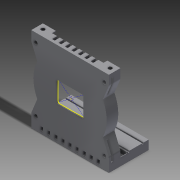
# Autodesk Inventor part: Nikon Base 02
Saved by Autodesk Inventor 2013 (Build 170138000, 138)
## iProperties
Created: 2014-04-13
Part Number: Nikon Base 02
Material: Generic
Document SubType Name: Modeling
Designer: spichelh
Density: 1 g/cm^3
Author: spichelh
Autodesk Inventor part; units mm, degrees
ref_plane "YZ Plane" through (0, 0, 0) normal (1, 0, 0) x (0, 1, 0)
ref_plane "XZ Plane" through (0, 0, 0) normal (0, 1, 0) x (-1, 0, 0)
ref_plane "XY Plane" through (0, 0, 0) normal (0, 0, 1) x (1, 0, 0)
sketch "Sketch1" plane through (0, 0, 0) normal (0, 0, 1) x (1, 0, 0)
  line L0 (0, -8.8929) -> (0, 44.5272) construction
  circle A0 centre (26.67, 24.765) radius 3.5 construction
  circle A1 centre (26.67, 24.765) radius 1.4
  line L1 (-0.1076, 0) -> (-29.2451, 0) construction
  line L2 (-21.59, -19.685) -> (-21.59, -28.575) construction
  circle A2 centre (-26.67, 24.765) radius 3.5 construction
  circle A3 centre (-26.67, 24.765) radius 1.4
  circle A4 centre (-26.67, -24.765) radius 1.4
  circle A5 centre (-26.67, -24.765) radius 3.5 construction
  circle A6 centre (26.67, -24.765) radius 1.4
  circle A7 centre (26.67, -24.765) radius 3.5 construction
  line L3 (-26.67, 24.765) -> (26.67, -24.765) construction
  line L4 (26.67, 24.765) -> (-26.67, -24.765) construction
  line L5 (-21.59, 19.685) -> (-21.59, 28.575) construction
  line L6 (21.59, -19.685) -> (21.59, -28.575) construction
  line L7 (21.59, 19.685) -> (21.59, 28.575) construction
  line L8 (-21.67, 30.575) -> (21.67, 30.575) construction
  line L9 (21.67, 30.575) -> (21.67, -25.765) construction
  line L10 (21.67, -25.765) -> (-21.67, -25.765) construction
  line L11 (-21.67, -25.765) -> (-21.67, 30.575) construction
  line L12 (-50.8, 28.575) -> (50.8, 28.575) construction
  line L13 (50.8, 28.575) -> (50.8, -28.575) construction
  line L14 (50.8, -28.575) -> (-50.8, -28.575) construction
  line L15 (-50.8, -28.575) -> (-50.8, 28.575) construction
  line L16 (-50.8, 28.575) -> (50.8, -28.575) construction
  line L17 (50.8, 28.575) -> (-50.8, -28.575) construction
  line L18 (-30.17, -29.575) -> (-30.17, -24.765)
  line L19 (30.17, -29.575) -> (30.17, -24.765)
  line L20 (-30.17, -29.575) -> (30.17, -29.575)
  line L21 (22.37, -28.575) -> (-22.37, -28.575)
  arc A8 (-29.9124, -23.447) -> (-30.17, -24.765) centre (-26.67, -24.765) ccw
  arc A9 (30.17, -24.765) -> (29.9124, -23.447) centre (26.67, -24.765) ccw
  circle A10 centre (26.67, 24.765) radius 1.4
  line L22 (30.17, 24.765) -> (30.17, 31.575)
  line L23 (-30.17, 31.575) -> (30.17, 31.575)
  line L24 (-30.17, 24.765) -> (-30.17, 31.575)
  line L25 (-22.37, 29.575) -> (22.37, 29.575)
  arc A11 (-30.17, 24.765) -> (-29.9124, 23.447) centre (-26.67, 24.765) ccw
  arc A12 (29.9124, 23.447) -> (30.17, 24.765) centre (26.67, 24.765) ccw
  circle A13 centre (0, 0) radius 28.5 construction
  line L26 (29.9124, -23.447) -> (25.5304, -12.6669)
  line L27 (29.9124, 23.447) -> (25.5304, 12.6669)
  arc A14 (25.5304, -12.6669) -> (25.5304, 12.6669) centre (0, 0) ccw
  line L28 (29.9124, 23.447) -> (26.67, 24.765) construction
  line L29 (-29.9124, -23.447) -> (-25.5304, -12.6669)
  line L30 (-29.9124, 23.447) -> (-25.5304, 12.6669)
  arc A15 (-25.5304, 12.6669) -> (-25.5304, -12.6669) centre (0, 0) ccw
  line L31 (22.37, 29.575) -> (22.37, -28.575)
  line L32 (-22.37, -28.575) -> (-22.37, 29.575)
  point P0 (0, 0)
  point P1 (0, 0)
  point P2 (0, 0)
  point P3 (24.8655, -21.7661)
  point P4 (0.1677, 29.575)
  point P5 (-23.17, 24.765)
  point P6 (-23.17, -24.765)
  point P7 (23.17, -24.765)
  point P8 (23.17, 24.765)
  point P9 (0, 0)
  point P10 (0, 0)
  point P11 (0, 0)
  dimension "d315" = 7
  dimension "d320" = 2.8
  dimension "d327" = 85
  dimension "d328" = 8.89
  dimension "d332" = 53.34
  dimension "d333" = 49.53
  dimension "d334" = 2.8
  dimension "d335" = 7
  dimension "d337" = 5.08
  dimension "d339" = 5
  dimension "d340" = 5
  dimension "d341" = 1
  dimension "d342" = 101.6
  dimension "d343" = 57.15
  dimension "d344" = 2
  dimension "d363" = 7
  dimension "d364" = 2.8
  dimension "d366" = 1
  dimension "d367" = 2
  dimension "d368" = 1
  dimension "d377" = 3.5
  dimension "d378" = 6.81
  dimension "d403" = 57
  dimension "d417" = 155
  dimension "d418" = 155
  dimension "d422" = 0.7
  dimension "d423" = 0.7
  constraints: 70 end point, 24 point on circle, 16 centre point, 15 symmetric about line, 7 coincident, 7 midpoint, 7 perpendicular, 6 parallel, 5 concentric, 5 tangent, 4 point on line, 3 horizontal, 2 horizontal alignment, 1 vertical alignment, 5 other
  measures "d315" diameter of A0
  measures "d320" diameter of A1
  measures "d328" distance of L2.start L2.end
  measures "d332" distance of A0.centre A2.centre
  measures "d333" distance of point (-26.67, -24.765) A2.centre
  measures "d334" diameter of A4
  measures "d335" diameter of A5
  measures "d337" distance from line of A4.centre L2
  measures "d339" distance from line of A0.centre L9
  measures "d340" distance from line of A2.centre L11
  measures "d341" distance from line of L10 A6.centre
  measures "d342" distance of L13.end L14.end
  measures "d343" distance of L12.end L13.end
  measures "d344" distance between parallel lines of L12 L8
  measures "d363" diameter of A2
  measures "d364" diameter of A3
  measures "d366" distance between parallel lines of L12 L25
  measures "d367" distance between parallel lines of L23 L25
  measures "d368" distance between parallel lines of L21 L20
  measures "d377" radius of A12
  measures "d378" distance of L22.start L22.end
  measures "d403" diameter of A13
  measures "d417" angle of L26 L3
  measures "d418" angle of L4 L27
  measures "d422" distance between parallel lines of L9 L31
  measures "d423" distance between parallel lines of L11 L32
extrude "Extrusion1" add sketch "Sketch1" along normal blind 9
sketch "Sketch14" plane through (0, 0, 9) normal (0, 0, 1) x (1, 0, 0)
  line L0 (50.88, 56.34) -> (5, 56.34) construction
  line L1 (-22.86, -0.81) -> (78.74, -0.81) construction
  line L2 (-22.86, 56.34) -> (-22.86, -0.81) construction
  line L3 (78.74, -0.81) -> (78.74, 56.34) construction
  circle A0 centre (26.67, 24.765) radius 1.4 projected
  arc A1 (-29.9124, -23.447) -> (-30.17, -24.765) centre (-26.67, -24.765) ccw projected
  line L4 (-30.17, -29.575) -> (30.17, -29.575) projected
  arc A2 (30.17, -24.765) -> (29.9124, -23.447) centre (26.67, -24.765) ccw projected
  line L5 (-27.94, 24.765) -> (26.67, -24.765) construction
  line L6 (-26.67, -24.765) -> (26.67, 24.765) construction
  circle A3 centre (0, 0) radius 23
  line L7 (27.3548, 30.2966) -> (-26.2048, 30.2966)
  line L8 (-26.67, -29.1989) -> (25.27, -29.1989)
  line L9 (30.17, 31.575) -> (-30.17, 31.575) projected
  line L10 (-26.2048, 30.2966) -> (-25.2211, 26.462)
  line L11 (-25.2211, 26.462) -> (-25.2211, 23)
  line L12 (-25.2211, 23) -> (-25.2211, 18.3922)
  line L13 (-25.2211, 18.3922) -> (-25.0819, 16.5883)
  line L14 (-25.1417, -26.7599) -> (-26.67, -29.1989)
  line L15 (25.27, -29.1989) -> (25.1417, -24.765)
  line L16 (25.1417, -24.765) -> (25.1912, -21.1)
  line L17 (25.1912, -21.1) -> (25.27, -15.2651)
  line L18 (25.27, -15.2651) -> (24.6585, -7.3445)
  line L19 (24.6585, -7.3445) -> (24.4818, 2.6027)
  line L20 (24.4818, 2.6027) -> (25.1533, 16.767)
  line L21 (25.1533, 16.767) -> (25.4405, 22.8257)
  line L22 (25.4405, 22.8257) -> (25.0053, 24.5219)
  line L23 (25.0053, 24.5219) -> (25.27, 26.707)
  line L24 (25.27, 26.707) -> (27.3548, 30.2966)
  line L25 (-30.17, 31.575) -> (-30.17, 24.765) projected
  line L26 (-25.1417, -26.7599) -> (-25.1417, -18.1825)
  line L27 (-25.1417, -18.1825) -> (-24.2585, 0.4493)
  line L28 (-24.2585, 0.4493) -> (-25.0819, 16.5883)
  dimension "d359" = 46
  constraints: 44 end point, 5 parallel, 3 collinear, 1 centre point, 1 midpoint, 1 perpendicular
  measures "d359" diameter of A3
extrude "Extrusion14" add sketch "Sketch14" against normal blind 2 contours L24 L23 L22 L21 L20 L19 L18 L17 L16 L15 L8 L14 L26 L27 L28 L13 L12 L11 L10 L7
sketch "Sketch17" plane through (0, 0, 7) normal (0, 0, -1) x (-1, 0, 0)
  line L0 (-9.4, 8.05) -> (9.4, 8.05)
  line L1 (10.4, 7.05) -> (10.4, -7.05)
  line L2 (9.4, -8.05) -> (-9.4, -8.05)
  line L3 (-10.4, -7.05) -> (-10.4, 7.05)
  line L4 (10.4, 8.05) -> (-10.4, -8.05) construction
  line L5 (10.4, -8.05) -> (-10.4, 8.05) construction
  circle A0 centre (0, 0) radius 23
  arc A1 (-9.4, 8.05) -> (-10.4, 7.05) centre (-9.4, 7.05) ccw
  arc A2 (-10.4, -7.05) -> (-9.4, -8.05) centre (-9.4, -7.05) ccw
  arc A3 (9.4, -8.05) -> (10.4, -7.05) centre (9.4, -7.05) ccw
  arc A4 (10.4, 7.05) -> (9.4, 8.05) centre (9.4, 7.05) ccw
  dimension "d111" = 20.8
  dimension "d112" = 16.1
  dimension "d115" = 1
  constraints: 12 end point, 8 point on circle, 8 point on line, 8 tangent, 5 centre point, 3 equal radius, 2 coincident, 2 parallel, 1 horizontal, 1 midpoint, 1 perpendicular
  measures "d111" distance of L5.start L4.end
  measures "d112" distance of L4.start L5.start
  measures "d115" radius of A1
extrude "Extrusion17" add sketch "Sketch17" against normal blind 2
sketch "Sketch26" plane through (0, 6, 0) normal (-1, 0, 0) x (0, 0, 1)
  line L0 (0, 43.53) -> (0, 0) projected
  line L1 (-1, 50.34) -> (0, 50.34) construction
  line L2 (-1, -6.81) -> (0, -6.81) construction
  line L3 (4, -6.81) -> (6, -6.81)
  line L4 (6, -6.81) -> (6, 50.34)
  line L5 (6, 50.34) -> (4, 50.34)
  line L6 (4, 50.34) -> (4, -6.81)
  point P0 (0, -6)
  dimension "d140" = 2
  dimension "d141" = 4
  constraints: 8 end point, 2 collinear, 2 parallel, 1 horizontal, 1 perpendicular
  measures "d140" distance of L5.end L4.end
  measures "d141" distance between parallel lines of L0 L6
extrude "Extrusion26" [suppressed]
sketch "Sketch27" plane through (55.88, 6, 0) normal (1, 0, 0) x (0, 0, -1)
  line L0 (1, -6.81) -> (0, -6.81) construction
  line L1 (1, 50.34) -> (0, 50.34) construction
  line L2 (-4, 50.34) -> (-6, 50.34)
  line L3 (-6, 50.34) -> (-6, -6.81)
  line L4 (-6, -6.81) -> (-4, -6.81)
  line L5 (-4, -6.81) -> (-4, 50.34)
  line L6 (0, -13) -> (0, -6) construction
  dimension "d146" = 2
  dimension "d147" = 4
  constraints: 8 end point, 2 collinear, 2 parallel, 1 horizontal, 1 perpendicular
  measures "d146" distance of L4.end L3.end
  measures "d147" distance between parallel lines of L6 L5
extrude "Extrusion27" [suppressed]
sketch "Sketch32" plane through (0, 0, 0) normal (0, 0, -1) x (-1, 0, 0)
  line L0 (-30.17, -34.575) -> (30.17, -34.575)
  line L1 (30.17, -34.575) -> (30.17, -28.575)
  line L2 (30.17, -28.575) -> (-30.17, -28.575)
  line L3 (-30.17, -28.575) -> (-30.17, -34.575)
  line L4 (30.17, -29.575) -> (-30.17, -29.575)
  circle A0 centre (-26.67, -24.765) radius 1.4 projected
  circle A1 centre (26.67, -24.765) radius 1.4 projected
  circle A2 centre (26.67, 24.765) radius 1.4 projected
  circle A3 centre (-26.67, 24.765) radius 1.4 projected
  line L5 (-30.17, 31.575) -> (30.17, 31.575) projected
  line L6 (-30.17, 24.765) -> (-30.17, 31.575) projected
  arc A4 (-29.9124, -23.447) -> (-30.17, -24.765) centre (-26.67, -24.765) ccw projected
  line L7 (-30.17, -29.575) -> (-30.17, -24.765) projected
  line L8 (30.17, -29.575) -> (-30.17, -29.575) projected
  line L9 (30.17, -24.765) -> (30.17, -29.575) projected
  arc A5 (30.17, -24.765) -> (29.9124, -23.447) centre (26.67, -24.765) ccw projected
  line L10 (0, -34.575) -> (0, -36.1591) construction
  line L11 (0, -31.3897) -> (0, -27.0731) construction
  line L12 (-30.17, -29.575) -> (-30.17, -24.765) projected
  arc A6 (29.9124, 23.447) -> (30.17, 24.765) centre (26.67, 24.765) ccw projected
  line L13 (30.17, 31.575) -> (30.17, 24.765) projected
  arc A7 (-30.17, 24.765) -> (-29.9124, 23.447) centre (-26.67, 24.765) ccw projected
  line L14 (25.5304, -12.6669) -> (29.9124, -23.447) projected
  arc A8 (25.5304, -12.6669) -> (25.5304, 12.6669) centre (0, 0) ccw projected
  line L15 (29.9124, 23.447) -> (25.5304, 12.6669) projected
  line L16 (-25.5304, 12.6669) -> (-29.9124, 23.447) projected
  arc A9 (-25.5304, 12.6669) -> (-25.5304, -12.6669) centre (0, 0) ccw projected
  line L17 (-29.9124, -23.447) -> (-25.5304, -12.6669) projected
  dimension "d180" = 6
  dimension "d432" = 1
  constraints: 14 end point, 3 collinear, 3 parallel, 1 horizontal, 1 midpoint, 1 perpendicular
  measures "d180" distance between parallel lines of L0 L2
  measures "d432" distance between parallel lines of L4 L2
extrude "Extrusion32" add sketch "Sketch32" along normal blind 22 and the other way blind 1.5 contours L3 L4 L1 L0 | L3 L2 L1 L4
sketch "Sketch35" plane through (-30.17, -34.575, -22) normal (0, -1, 0) x (1, 0, 0)
  line L0 (60.34, 33) -> (0, 33)
  line L1 (0, 33) -> (60.34, 0) construction
  line L2 (60.34, 33) -> (0, 0) construction
  line L3 (30.17, 16.5) -> (30.17, -14.8721) construction
  circle A0 centre (30.17, 6.5) radius 3.175
  circle A1 centre (30.17, 18.5) radius 3.175
  line L4 (0, 23.5) -> (60.34, 23.5) projected
  dimension "d194" = 6.35
  dimension "d195" = 10
  dimension "d196" = 6.35
  dimension "d197" = 2
  dimension "d369" = 5
  constraints: 8 end point, 2 centre point, 2 point on line, 2 vertical alignment, 1 horizontal, 1 midpoint, 1 perpendicular
  measures "d194" diameter of A0
  measures "d195" distance of L3.start A0.centre
  measures "d196" diameter of A1
  measures "d197" distance of L3.start A1.centre
  measures "d369" distance from line of A1.centre L4
extrude "Extrusion34" cut sketch "Sketch35" against normal blind 10
sketch "Sketch37" plane through (52.88, -28.575, 0) normal (0, 1, 0) x (1, 0, 0)
  line L0 (-49.88, -1.5) -> (-49.88, 0) projected
  line L1 (3, -1.5) -> (-52.88, -1.5) projected
  line L2 (0, -1.5) -> (-49.88, -1.5)
  line L3 (-49.88, -1.5) -> (-49.88, 0)
  line L4 (-49.88, 0) -> (0, 0)
  line L5 (0, 0) -> (0, -1.5)
  constraints: 8 end point, 2 parallel, 1 horizontal, 1 perpendicular
extrude "Extrusion36" [suppressed]
sketch "Sketch38" plane through (0, 0, 7) normal (0, 0, -1) x (-1, 0, 0)
  arc A0 (-10.4, -7.05) -> (-9.4, -8.05) centre (-9.4, -7.05) ccw projected
  line L0 (-10.4, -7.05) -> (-10.4, 7.05) projected
  arc A1 (-9.4, 8.05) -> (-10.4, 7.05) centre (-9.4, 7.05) ccw projected
  line L1 (-9.4, 8.05) -> (9.4, 8.05) projected
  arc A2 (10.4, 7.05) -> (9.4, 8.05) centre (9.4, 7.05) ccw projected
  line L2 (10.4, 7.05) -> (10.4, -7.05) projected
  arc A3 (9.4, -8.05) -> (10.4, -7.05) centre (9.4, -7.05) ccw projected
  line L3 (9.4, -8.05) -> (-9.4, -8.05) projected
  line L4 (9.4, 7.05) -> (-9.4, -7.05) construction
  line L5 (9.4, -7.05) -> (-9.4, 7.05) construction
  line L6 (-21.665, 19.44) -> (21.665, 19.44)
  line L7 (21.665, 19.44) -> (21.665, -19.44)
  line L8 (21.665, -19.44) -> (-21.665, -19.44)
  line L9 (-21.665, -19.44) -> (-21.665, 19.44)
  line L10 (21.665, -19.44) -> (-21.665, 19.44) construction
  line L11 (-21.665, -19.44) -> (21.665, 19.44) construction
  point P0 (0, 0)
  point P1 (0, 0)
  dimension "d209" = 38.88
  dimension "d211" = 43.33
  constraints: 16 end point, 3 midpoint, 2 parallel, 1 horizontal, 1 perpendicular
  measures "d209" distance of L8.end L6.start
  measures "d211" distance of L6.start L6.end
extrude "Extrusion37" cut sketch "Sketch38" against normal blind 1
sketch "Sketch39" plane through (0, 0, 8) normal (0, 0, -1) x (-1, 0, 0)
  line L0 (-9.4, -8.05) -> (9.4, -8.05) projected
  arc A0 (-10.4, -7.05) -> (-9.4, -8.05) centre (-9.4, -7.05) ccw projected
  line L1 (-10.4, 7.05) -> (-10.4, -7.05) projected
  arc A1 (-9.4, 8.05) -> (-10.4, 7.05) centre (-9.4, 7.05) ccw projected
  line L2 (9.4, 8.05) -> (-9.4, 8.05) projected
  arc A2 (10.4, 7.05) -> (9.4, 8.05) centre (9.4, 7.05) ccw projected
  line L3 (10.4, -7.05) -> (10.4, 7.05) projected
  arc A3 (9.4, -8.05) -> (10.4, -7.05) centre (9.4, -7.05) ccw projected
  line L4 (-21.665, 19.44) -> (21.665, 19.44) projected
  line L5 (-21.665, -19.44) -> (-21.665, 19.44) projected
  line L6 (21.665, -19.44) -> (-21.665, -19.44) projected
  line L7 (21.665, 19.44) -> (21.665, -19.44) projected
  line L8 (9.4, 7.05) -> (-9.4, -7.05) construction
  line L9 (-9.4, 7.05) -> (9.4, -7.05) construction
  point P0 (0, 0)
  point P1 (0, 0)
  constraints: 4 end point, 1 midpoint
sketch "Sketch40" plane through (0, 0, 9) normal (0, 0, 1) x (1, 0, 0)
  line L0 (-20, 31.575) -> (20, 31.575)
  line L1 (20, 31.575) -> (20, 33.575)
  line L2 (20, 33.575) -> (-20, 33.575)
  line L3 (-20, 33.575) -> (-20, 31.575)
  line L4 (30.17, 31.575) -> (-30.17, 31.575) projected
  line L5 (0, 33.575) -> (0, 37.7765) construction
  line L6 (0, 31.575) -> (0, 28.075) construction
  dimension "d216" = 2
  dimension "d217" = 40
  constraints: 12 end point, 3 collinear, 2 midpoint, 2 parallel, 1 horizontal, 1 perpendicular, 1 vertical
  measures "d216" distance of L2.end L0.start
  measures "d217" distance between parallel lines of L3 L1
extrude "Extrusion38" [suppressed]
sketch "Sketch43" plane through (-30.17, 31.575, 0) normal (0, 1, 0) x (1, 0, 0)
  line L0 (47.17, 21) -> (13.17, 21)
  line L1 (13.17, 26) -> (13.17, 21)
  line L2 (47.17, 26) -> (13.17, 26)
  line L3 (47.17, 26) -> (47.17, 21)
  line L4 (14.17, 27) -> (16.17, 27)
  line L5 (16.17, 27) -> (16.17, 22)
  line L6 (16.17, 22) -> (14.17, 22)
  line L7 (14.17, 22) -> (14.17, 27)
  line L8 (19.17, 27) -> (21.17, 27)
  line L9 (21.17, 27) -> (21.17, 22)
  line L10 (21.17, 22) -> (19.17, 22)
  line L11 (19.17, 22) -> (19.17, 27)
  line L12 (24.17, 27) -> (26.17, 27)
  line L13 (26.17, 27) -> (26.17, 22)
  line L14 (26.17, 22) -> (24.17, 22)
  line L15 (24.17, 22) -> (24.17, 27)
  line L16 (29.17, 27) -> (31.17, 27)
  line L17 (31.17, 27) -> (31.17, 22)
  line L18 (31.17, 22) -> (29.17, 22)
  line L19 (29.17, 22) -> (29.17, 27)
  line L20 (34.17, 27) -> (36.17, 27)
  line L21 (36.17, 27) -> (36.17, 22)
  line L22 (36.17, 22) -> (34.17, 22)
  line L23 (34.17, 22) -> (34.17, 27)
  line L24 (39.17, 27) -> (41.17, 27)
  line L25 (41.17, 27) -> (41.17, 22)
  line L26 (41.17, 22) -> (39.17, 22)
  line L27 (39.17, 22) -> (39.17, 27)
  line L28 (44.17, 27) -> (46.17, 27)
  line L29 (46.17, 27) -> (46.17, 22)
  line L30 (46.17, 22) -> (44.17, 22)
  line L31 (44.17, 22) -> (44.17, 27)
  line L32 (10.17, 39.892) -> (10.17, -9)
  line L33 (50.17, 39.3269) -> (50.17, -9)
  line L34 (10.17, 10) -> (50.17, 10) construction
  line L35 (14.17, -7) -> (16.17, -7)
  line L36 (16.17, -7) -> (16.17, -2)
  line L37 (16.17, -2) -> (14.17, -2)
  line L38 (14.17, -2) -> (14.17, -7)
  line L39 (21.17, -7) -> (21.17, -2)
  line L40 (19.17, -7) -> (21.17, -7)
  line L41 (21.17, -2) -> (19.17, -2)
  line L42 (26.17, -7) -> (26.17, -2)
  line L43 (24.17, -7) -> (26.17, -7)
  line L44 (24.17, -2) -> (24.17, -7)
  line L45 (26.17, -2) -> (24.17, -2)
  line L46 (31.17, -7) -> (31.17, -2)
  line L47 (29.17, -7) -> (31.17, -7)
  line L48 (29.17, -2) -> (29.17, -7)
  line L49 (31.17, -2) -> (29.17, -2)
  line L50 (36.17, -7) -> (36.17, -2)
  line L51 (34.17, -7) -> (36.17, -7)
  line L52 (34.17, -2) -> (34.17, -7)
  line L53 (36.17, -2) -> (34.17, -2)
  line L54 (41.17, -7) -> (41.17, -2)
  line L55 (39.17, -7) -> (41.17, -7)
  line L56 (39.17, -2) -> (39.17, -7)
  line L57 (41.17, -2) -> (39.17, -2)
  line L58 (46.17, -7) -> (46.17, -2)
  line L59 (44.17, -7) -> (46.17, -7)
  line L60 (44.17, -2) -> (44.17, -7)
  line L61 (46.17, -2) -> (44.17, -2)
  line L62 (19.17, -2) -> (19.17, -7)
  line L63 (50.17, -9) -> (10.17, -9)
  line L64 (50.17, -9) -> (40, -9)
  line L65 (60.34, -9) -> (0, -9) projected
  line L66 (60.34, 0) -> (60.34, -9) projected
  line L67 (30.17, -9) -> (30.17, -4.5) construction
  line L68 (30.17, -9) -> (30.17, 3.8143) construction
  point P0 (0, 27)
  point P1 (50.17, 39.3269)
  dimension "d233" = 1
  dimension "d234" = 1
  dimension "d235" = 2
  dimension "d236" = 1
  dimension "d239" = 5
  dimension "d295" = 3
  dimension "d296" = 3
  dimension "d297" = 1
  dimension "d298" = 5
  dimension "d299" = 19
  dimension "d370" = 2
  dimension "d371" = 4
  dimension "d372" = 4
  dimension "d447" = 40
  constraints: 132 end point, 28 symmetric about line, 4 collinear, 3 horizontal, 3 parallel, 2 midpoint, 1 perpendicular, 1 point on line, 52 other
  measures "d233" distance between parallel lines of L2 L4
  measures "d234" distance between parallel lines of L0 L6
  measures "d235" distance between parallel lines of L7 L5
  measures "d236" distance between parallel lines of L7 L1
  measures "d239" distance of L4.end L9.start
  measures "d295" distance between parallel lines of L32 L1
  measures "d297" distance between parallel lines of L3 L29
  measures "d298" distance between parallel lines of L8 L10
  measures "d299" distance between parallel lines of L63 L34
  measures "d370" distance between parallel lines of L64 L40
  measures "d372" distance between parallel lines of L32 L38
extrude "Extrusion41" cut sketch "Sketch43" against normal blind 5 contours L29 L30 L31 L2 | L2 L31 L28 L29 | L7 L4 L5 L2 | L2 L5 L6 L7 | L25 L26 L27 L2 | L2 L27 L24 L25 | L11 L8 L9 L2 | L2 L9 L10 L11 | L21 L22 L23 L2 | L2 L23 L20 L21 | L15 L12 L13 L2 | L2 L13 L14 L15 | L17 L18 L19 L2 | L2 L19 L16 L17 | L38 L37 L36 L35 | L40 L62 L41 L39 | L43 L44 L45 L42 | L47 L48 L49 L46 | L51 L52 L53 L50 | L55 L56 L57 L54 | L59 L60 L61 L58
sketch "Sketch44" plane through (-24.8655, -28.575, 0) normal (0, 1, 0) x (1, 0, 0)
  line L0 (49.88, -7.5) -> (0, -7.5)
  line L1 (0, -7.5) -> (0, 0)
  line L2 (0, 0) -> (49.88, 0)
  line L3 (49.88, -7.5) -> (49.88, 0)
  line L4 (2, -1) -> (4, -1)
  line L5 (4, -1) -> (4, -6.5)
  line L6 (4, -6.5) -> (2, -6.5)
  line L7 (2, -6.5) -> (2, -1)
  line L8 (7.5, -1) -> (9.5, -1)
  line L9 (9.5, -1) -> (9.5, -6.5)
  line L10 (9.5, -6.5) -> (7.5, -6.5)
  line L11 (7.5, -6.5) -> (7.5, -1)
  line L12 (13, -1) -> (15, -1)
  line L13 (15, -1) -> (15, -6.5)
  line L14 (15, -6.5) -> (13, -6.5)
  line L15 (13, -6.5) -> (13, -1)
  line L16 (18.5, -1) -> (20.5, -1)
  line L17 (20.5, -1) -> (20.5, -6.5)
  line L18 (20.5, -6.5) -> (18.5, -6.5)
  line L19 (18.5, -6.5) -> (18.5, -1)
  line L20 (24, -1) -> (26, -1)
  line L21 (26, -1) -> (26, -6.5)
  line L22 (26, -6.5) -> (24, -6.5)
  line L23 (24, -6.5) -> (24, -1)
  line L24 (29.5, -1) -> (31.5, -1)
  line L25 (31.5, -1) -> (31.5, -6.5)
  line L26 (31.5, -6.5) -> (29.5, -6.5)
  line L27 (29.5, -6.5) -> (29.5, -1)
  line L28 (35, -1) -> (37, -1)
  line L29 (37, -1) -> (37, -6.5)
  line L30 (37, -6.5) -> (35, -6.5)
  line L31 (35, -6.5) -> (35, -1)
  line L32 (40.5, -1) -> (42.5, -1)
  line L33 (42.5, -1) -> (42.5, -6.5)
  line L34 (42.5, -6.5) -> (40.5, -6.5)
  line L35 (40.5, -6.5) -> (40.5, -1)
  line L36 (46, -1) -> (48, -1)
  line L37 (48, -1) -> (48, -6.5)
  line L38 (48, -6.5) -> (46, -6.5)
  line L39 (46, -6.5) -> (46, -1)
  point P0 (0, -9)
  dimension "d247" = 1
  dimension "d248" = 1
  dimension "d249" = 2
  dimension "d250" = 2
  dimension "d253" = 5.5
  dimension "d260" = 1.88
  constraints: 80 end point, 2 horizontal, 2 parallel, 1 perpendicular, 64 other
  measures "d247" distance between parallel lines of L2 L4
  measures "d248" distance between parallel lines of L0 L6
  measures "d249" distance between parallel lines of L7 L5
  measures "d250" distance between parallel lines of L1 L7
  measures "d253" distance of L4.end L9.start
  measures "d260" distance between parallel lines of L37 L3
extrude "Extrusion42" cut sketch "Sketch44" against normal blind 5 contours L4 L5 L6 L7 | L8 L9 L10 L11 | L12 L13 L14 L15 | L16 L17 L18 L19 | L20 L21 L22 L23 | L24 L25 L26 L27 | L28 L29 L30 L31 | L32 L33 L34 L35 | L36 L37 L38 L39
sketch "Sketch46" plane through (-20, 33.575, 15) normal (0, 1, 0) x (1, 0, 0)
  circle A0 centre (4, 36) radius 1.7
  circle A1 centre (36, 36) radius 1.7
  line L0 (36, 36) -> (4, 36) construction
  circle A2 centre (36, 4) radius 1.7
  line L1 (0, 40) -> (0, 0) projected
  line L2 (40, 0) -> (0, 0) projected
  line L3 (40, 40) -> (40, 0) projected
  line L4 (0, 40) -> (40, 40) projected
  line L5 (40, 20) -> (0, 20) construction
  line L6 (20, 40) -> (20, 0) construction
  line L7 (36, 4) -> (36, 36) construction
  circle A3 centre (4, 4) radius 1.7
  point P0 (20, 36)
  point P1 (36, 20)
  dimension "d275" = 3.4
  dimension "d277" = 3.4
  dimension "d278" = 32
  dimension "d279" = 32
  dimension "d294" = 3.4
  constraints: 8 end point, 6 midpoint, 4 centre point, 2 point on line, 1 horizontal, 1 symmetric about line, 1 other
  measures "d275" diameter of A0
  measures "d277" diameter of A1
  measures "d278" distance of L0.start L0.end
  measures "d279" distance of L7.start L0.start
  measures "d294" diameter of A2
extrude "Extrusion44" [suppressed]
sketch "Sketch49" plane through (0, 0, 0) normal (0, 0, -1) x (-1, 0, 0)
  line L0 (0, 55.53) -> (0, 58.53) projected
  line L1 (-55.88, 58.53) -> (0, 58.53)
  line L2 (0, 58.53) -> (0, 56.53)
  line L3 (0, 56.53) -> (-55.88, 56.53)
  line L4 (-55.88, 56.53) -> (-55.88, 58.53)
  constraints: 8 end point, 2 parallel, 1 horizontal, 1 perpendicular, 1 point on line
extrude "Extrusion46" [suppressed]
sketch "Sketch51" plane through (0, 0, 7) normal (0, 0, -1) x (-1, 0, 0)
  line L0 (21.665, -19.44) -> (-21.665, -19.44) projected
  line L1 (-3, -2.5) -> (-52.88, -2.5) projected
  line L2 (-37.44, -2.5) -> (-35.44, -2.5)
  line L3 (-35.44, -2.5) -> (-35.44, 0.5)
  line L4 (-35.44, 0.5) -> (-37.44, 0.5)
  line L5 (-37.44, 0.5) -> (-37.44, -2.5)
  line L6 (-27.94, -2.5) -> (-27.94, -19.44) construction
  line L7 (-31.94, -2.5) -> (-29.94, -2.5)
  line L8 (-29.94, -2.5) -> (-29.94, 0.5)
  line L9 (-29.94, 0.5) -> (-31.94, 0.5)
  line L10 (-31.94, 0.5) -> (-31.94, -2.5)
  line L11 (-26.44, -2.5) -> (-24.44, -2.5)
  line L12 (-24.44, -2.5) -> (-24.44, 0.5)
  line L13 (-24.44, 0.5) -> (-26.44, 0.5)
  line L14 (-26.44, 0.5) -> (-26.44, -2.5)
  line L15 (-20.94, -2.5) -> (-18.94, -2.5)
  line L16 (-18.94, -2.5) -> (-18.94, 0.5)
  line L17 (-18.94, 0.5) -> (-20.94, 0.5)
  line L18 (-20.94, 0.5) -> (-20.94, -2.5)
  point P0 (0, 0)
  dimension "d300" = 0
  dimension "d301" = 2
  dimension "d302" = 3
  dimension "d303" = 15
  dimension "d308" = 5.5
  constraints: 34 end point, 2 horizontal, 2 parallel, 1 midpoint, 1 perpendicular, 1 point on line, 24 other
  measures "d300" distance between parallel lines of L2 L1
  measures "d301" distance of L2.start L2.end
  measures "d302" distance between parallel lines of L4 L2
  measures "d303" diameter of L3 L6
  measures "d308" distance of L3.end L9.start
extrude "Extrusion48" [suppressed]
sketch "Sketch52" plane through (0, 0, 1.5) normal (0, 0, 1) x (1, 0, 0)
  line L0 (-30.17, -34.575) -> (30.17, -34.575) projected
  line L1 (30.17, -34.575) -> (30.17, -29.575) projected
  line L2 (-30.17, -29.575) -> (30.17, -29.575) projected
  line L3 (-30.17, -29.575) -> (-30.17, -34.575) projected
  line L4 (-30.17, -34.575) -> (30.17, -34.575) projected
  line L5 (30.17, -34.575) -> (30.17, -29.575) projected
  line L6 (-30.17, -29.575) -> (-22.8655, -29.575) projected
  line L7 (-30.17, -29.575) -> (-30.17, -34.575) projected
  line L8 (15.6345, -33.575) -> (15.6345, -29.575) projected
  line L9 (12.1345, -29.575) -> (15.6345, -29.575) projected
  line L10 (12.1345, -29.575) -> (12.1345, -33.575) projected
  line L11 (12.1345, -33.575) -> (10.1345, -33.575) projected
  line L12 (10.1345, -33.575) -> (10.1345, -29.575) projected
  line L13 (6.6345, -29.575) -> (10.1345, -29.575) projected
  line L14 (6.6345, -29.575) -> (6.6345, -33.575) projected
  line L15 (6.6345, -33.575) -> (4.6345, -33.575) projected
  line L16 (4.6345, -33.575) -> (4.6345, -29.575) projected
  line L17 (1.1345, -29.575) -> (4.6345, -29.575) projected
  line L18 (1.1345, -29.575) -> (1.1345, -33.575) projected
  line L19 (1.1345, -33.575) -> (-0.8655, -33.575) projected
  line L20 (-0.8655, -33.575) -> (-0.8655, -29.575) projected
  line L21 (-4.3655, -29.575) -> (-0.8655, -29.575) projected
  line L22 (-4.3655, -29.575) -> (-4.3655, -33.575) projected
  line L23 (-4.3655, -33.575) -> (-6.3655, -33.575) projected
  line L24 (-6.3655, -33.575) -> (-6.3655, -29.575) projected
  line L25 (-9.8655, -29.575) -> (-9.8655, -33.575) projected
  line L26 (-9.8655, -33.575) -> (-11.8655, -33.575) projected
  line L27 (-11.8655, -33.575) -> (-11.8655, -29.575) projected
  line L28 (-15.3655, -29.575) -> (-11.8655, -29.575) projected
  line L29 (-15.3655, -29.575) -> (-15.3655, -33.575) projected
  line L30 (-15.3655, -33.575) -> (-17.3655, -33.575) projected
  line L31 (-17.3655, -33.575) -> (-17.3655, -29.575) projected
  line L32 (-20.8655, -29.575) -> (-17.3655, -29.575) projected
  line L33 (-20.8655, -29.575) -> (-20.8655, -33.575) projected
  line L34 (-20.8655, -33.575) -> (-22.8655, -33.575) projected
  line L35 (-22.8655, -33.575) -> (-22.8655, -29.575) projected
  line L36 (23.1345, -29.575) -> (30.17, -29.575) projected
  line L37 (23.1345, -29.575) -> (23.1345, -33.575) projected
  line L38 (23.1345, -33.575) -> (21.1345, -33.575) projected
  line L39 (21.1345, -33.575) -> (21.1345, -29.575) projected
  line L40 (17.6345, -29.575) -> (21.1345, -29.575) projected
  line L41 (17.6345, -29.575) -> (17.6345, -33.575) projected
  line L42 (17.6345, -33.575) -> (15.6345, -33.575) projected
  line L43 (-9.8655, -29.575) -> (-6.3655, -29.575) projected
  point P0 (0, 0)
extrude "Extrusion49" add sketch "Sketch52" along normal blind 7.5
sketch "Sketch54" plane through (0, 0, 9) normal (0, 0, 1) x (1, 0, 0)
  line L0 (-30.17, -24.765) -> (-30.17, -34.575) projected
  line L1 (-30.17, -34.575) -> (30.17, -34.575) projected
  line L2 (30.17, -34.575) -> (30.17, -24.765) projected
  line L3 (-23, -29.575) -> (-21, -29.575)
  line L4 (-21, -29.575) -> (-21, -32.575)
  line L5 (-21, -32.575) -> (-23, -32.575)
  line L6 (-23, -32.575) -> (-23, -29.575)
  line L7 (-17.5, -29.575) -> (-15.5, -29.575)
  line L8 (-15.5, -29.575) -> (-15.5, -32.575)
  line L9 (-15.5, -32.575) -> (-17.5, -32.575)
  line L10 (-17.5, -32.575) -> (-17.5, -29.575)
  line L11 (-12, -29.575) -> (-10, -29.575)
  line L12 (-10, -29.575) -> (-10, -32.575)
  line L13 (-10, -32.575) -> (-12, -32.575)
  line L14 (-12, -32.575) -> (-12, -29.575)
  line L15 (-6.5, -29.575) -> (-4.5, -29.575)
  line L16 (-4.5, -29.575) -> (-4.5, -32.575)
  line L17 (-4.5, -32.575) -> (-6.5, -32.575)
  line L18 (-6.5, -32.575) -> (-6.5, -29.575)
  line L19 (-1, -29.575) -> (1, -29.575)
  line L20 (1, -29.575) -> (1, -32.575)
  line L21 (1, -32.575) -> (-1, -32.575)
  line L22 (-1, -32.575) -> (-1, -29.575)
  line L23 (4.5, -29.575) -> (6.5, -29.575)
  line L24 (6.5, -29.575) -> (6.5, -32.575)
  line L25 (6.5, -32.575) -> (4.5, -32.575)
  line L26 (4.5, -32.575) -> (4.5, -29.575)
  line L27 (10, -29.575) -> (12, -29.575)
  line L28 (12, -29.575) -> (12, -32.575)
  line L29 (12, -32.575) -> (10, -32.575)
  line L30 (10, -32.575) -> (10, -29.575)
  line L31 (15.5, -29.575) -> (17.5, -29.575)
  line L32 (17.5, -29.575) -> (17.5, -32.575)
  line L33 (17.5, -32.575) -> (15.5, -32.575)
  line L34 (15.5, -32.575) -> (15.5, -29.575)
  line L35 (21, -29.575) -> (23, -29.575)
  line L36 (23, -29.575) -> (23, -32.575)
  line L37 (23, -32.575) -> (21, -32.575)
  line L38 (21, -32.575) -> (21, -29.575)
  point P0 (0, 0)
  point P1 (-30.17, -29.575)
  point P2 (30.17, -29.575)
  dimension "d379" = 2
  dimension "d380" = 3
  dimension "d383" = 5.5
  dimension "d388" = 2
  dimension "d389" = 7.17
  dimension "d390" = 7.17
  constraints: 72 end point, 2 horizontal, 2 parallel, 1 collinear, 1 perpendicular, 63 other
  measures "d379" distance of L4.end L5.end
  measures "d380" distance of L3.end L4.end
  measures "d383" distance of L3.start L7.start
  measures "d388" distance between parallel lines of L5 L1
  measures "d389" distance between parallel lines of L0 L6
  measures "d390" distance between parallel lines of L2 L36
extrude "Extrusion51" cut sketch "Sketch54" against normal blind 8
sketch "Sketch55" plane through (0, 0, 0) normal (0, 0, -1) x (-1, 0, 0)
  line L0 (-20, 31.575) -> (20, 31.575) projected
  line L1 (-20, 31.575) -> (20, 31.575)
  line L2 (20, 31.575) -> (20, 29.575)
  line L3 (20, 29.575) -> (-20, 29.575)
  line L4 (-20, 29.575) -> (-20, 31.575)
  line L5 (-20, 33.575) -> (-20, 31.575) projected
  line L6 (20, 31.575) -> (20, 33.575) projected
  point P0 (-16, 31.575)
  point P1 (0, 0)
  dimension "d395" = 2
  constraints: 8 end point, 2 collinear, 2 parallel, 1 horizontal, 1 perpendicular, 1 point on line
  measures "d395" distance of L3.end L1.start
extrude "Extrusion52" cut sketch "Sketch55" against normal blind 3
sketch "Sketch56" plane through (0, 0, 0) normal (0, 0, -1) x (-1, 0, 0)
  line L0 (-20, 29.575) -> (-20, 31.575) projected
  line L1 (-30.17, 31.575) -> (-20, 31.575) projected
  line L2 (20, 29.575) -> (22.37, 29.575) projected
  line L3 (-22, 30.575) -> (21.185, 30.575)
  line L4 (21.185, 30.575) -> (21.185, 29.575)
  line L5 (21.185, 29.575) -> (-22, 29.575)
  line L6 (-22, 29.575) -> (-22, 30.575)
  point P0 (23.17, 29.575)
  point P1 (0, 0)
  dimension "d397" = 2
  dimension "d398" = 1
  constraints: 8 end point, 2 parallel, 1 horizontal, 1 midpoint, 1 perpendicular
  measures "d397" distance between parallel lines of L6 L0
  measures "d398" distance between parallel lines of L1 L3
extrude "Extrusion53" cut sketch "Sketch56" against normal blind 3
sketch "Sketch57" plane through (0, 0, 0) normal (0, 0, -1) x (-1, 0, 0)
  line L0 (-23.4203, 26.5752) -> (-29.9199, 26.5748) construction
  line L1 (-29.9199, 26.5748) -> (-30.1702, 28.5748) construction
  line L2 (-30.1702, 28.5748) -> (-30.1703, 29.9748) construction
  arc A0 (-29.5703, 30.5748) -> (-30.1703, 29.9748) centre (-29.5703, 29.9748) ccw construction
  line L3 (-29.5703, 30.5748) -> (-23.7703, 30.5752) construction
  arc A1 (-23.1703, 29.9752) -> (-23.7703, 30.5752) centre (-23.7703, 29.9752) ccw construction
  line L4 (-23.1703, 29.9752) -> (-23.1702, 28.5752) construction
  line L5 (-23.1702, 28.5752) -> (-23.4203, 26.5752) construction
  line L6 (20, 31.575) -> (20, 30.575) projected
  line L7 (0, 19.4123) -> (0, 6.0259) construction
  line L8 (30.17, 31.575) -> (-20, 31.575) projected
  line L9 (-29.0703, 30.6752) -> (-24.2699, 30.6752)
  line L10 (-29.5075, 26.4752) -> (-23.8327, 26.4752)
  line L11 (-29.5075, 26.4752) -> (-29.7703, 28.5748)
  line L12 (-29.7703, 29.9752) -> (-29.7703, 28.5748)
  arc A2 (-29.0703, 30.6752) -> (-29.7703, 29.9752) centre (-29.0703, 29.9752) ccw
  line L13 (-30.1702, 28.5748) -> (-29.2504, 28.5748) construction
  line L14 (-26.6701, 26.575) -> (-26.6701, 28.0459) construction
  line L15 (-23.8327, 26.4752) -> (-23.5699, 28.5748)
  line L16 (-23.5699, 29.9752) -> (-23.5699, 28.5748)
  arc A3 (-23.5699, 29.9752) -> (-24.2699, 30.6752) centre (-24.2699, 29.9752) ccw
  line L17 (29.0703, 30.6752) -> (24.2699, 30.6752)
  line L18 (29.5075, 26.4752) -> (23.8327, 26.4752)
  line L19 (29.5075, 26.4752) -> (29.7703, 28.5748)
  line L20 (29.7703, 29.9752) -> (29.7703, 28.5748)
  arc A4 (29.7703, 29.9752) -> (29.0703, 30.6752) centre (29.0703, 29.9752) ccw
  arc A5 (24.2699, 30.6752) -> (23.5699, 29.9752) centre (24.2699, 29.9752) ccw
  line L21 (23.5699, 29.9752) -> (23.5699, 28.5748)
  line L22 (23.8327, 26.4752) -> (23.5699, 28.5748)
  arc A6 (26.1996, -11.2173) -> (26.1996, 11.2173) centre (0, 0) ccw projected
  line L23 (30.17, 31.575) -> (30.17, 24.765) projected
  line L24 (0, 0) -> (-8.9535, 0) construction
  line L25 (-29.0703, -30.6752) -> (-24.2699, -30.6752)
  line L26 (-29.5075, -26.4752) -> (-23.8327, -26.4752)
  line L27 (-29.5075, -26.4752) -> (-29.7703, -28.5748)
  line L28 (-29.7703, -29.9752) -> (-29.7703, -28.5748)
  arc A7 (-29.7703, -29.9752) -> (-29.0703, -30.6752) centre (-29.0703, -29.9752) ccw
  arc A8 (-24.2699, -30.6752) -> (-23.5699, -29.9752) centre (-24.2699, -29.9752) ccw
  line L29 (-23.5699, -29.9752) -> (-23.5699, -28.5748)
  line L30 (-23.8327, -26.4752) -> (-23.5699, -28.5748)
  line L31 (23.8327, -26.4752) -> (23.5699, -28.5748)
  line L32 (23.5699, -29.9752) -> (23.5699, -28.5748)
  arc A9 (23.5699, -29.9752) -> (24.2699, -30.6752) centre (24.2699, -29.9752) ccw
  line L33 (29.0703, -30.6752) -> (24.2699, -30.6752)
  arc A10 (29.0703, -30.6752) -> (29.7703, -29.9752) centre (29.0703, -29.9752) ccw
  line L34 (29.7703, -29.9752) -> (29.7703, -28.5748)
  line L35 (29.5075, -26.4752) -> (29.7703, -28.5748)
  line L36 (29.5075, -26.4752) -> (23.8327, -26.4752)
  dimension "d408" = 0.1
  dimension "d410" = 0.1
  dimension "d411" = 0.4
  dimension "d412" = 0.7
  dimension "d413" = 6.2004
  dimension "d414" = 0.6
  constraints: 68 end point, 35 symmetric about line, 20 point on circle, 10 centre point, 4 parallel, 4 perpendicular, 2 tangent, 1 midpoint, 1 point on line, 25 other
  measures "d408" distance from line of L3.end L9
  measures "d410" distance from line of L0.start L10
  measures "d411" distance from line of L2.end L12
  measures "d412" radius of A2
  measures "d413" distance between parallel lines of L12 L16
  measures "d414" radius of A0
extrude "Extrusion54" cut sketch "Sketch57" along normal blind 5 and the other way blind 1.1
ref_plane "Work Plane1" through (0, 0, 7) normal (0, 0, -1) x (-1, 0, 0)
sketch "Sketch58" plane through (0, 0, 7) normal (0, 0, -1) x (-1, 0, 0)
  line L0 (-50.8002, 28.5736) -> (-22.8602, 28.5752)
  circle A0 centre (-26.67, 24.765) radius 1.4
  line L1 (-22.8602, 28.5752) -> (-22.8601, 26.0352)
  line L2 (-22.8601, 26.0352) -> (-24.1301, 26.0351)
  line L3 (-24.1301, 26.0351) -> (-24.1299, 23.4951)
  line L4 (-24.1299, 23.4951) -> (-22.8599, 23.4952)
  line L5 (-22.8599, 23.4952) -> (-22.8597, 19.6852)
  arc A1 (-22.8597, 19.6852) -> (-22.8575, -19.6848) centre (-1.3762, 0.0014) ccw
  line L6 (-22.8575, -19.6848) -> (-22.8573, -23.4948)
  line L7 (-22.8573, -23.4948) -> (-24.1273, -23.4949)
  line L8 (-24.1273, -23.4949) -> (-24.1271, -26.0349)
  line L9 (-24.1271, -26.0349) -> (-22.8571, -26.0348)
  line L10 (-22.8571, -26.0348) -> (-22.857, -28.5748)
  line L11 (-22.857, -28.5748) -> (-50.797, -28.5764)
  circle A2 centre (-26.6672, -24.765) radius 1.4
  line L12 (24.1301, 23.4979) -> (24.1302, 20.9579)
  line L13 (22.8601, 23.4978) -> (24.1301, 23.4979)
  line L14 (22.8598, 28.5778) -> (22.8601, 23.4978)
  line L15 (24.1302, 20.9579) -> (22.8602, 20.9578)
  line L16 (22.8602, 20.9578) -> (22.8603, 19.6878)
  arc A3 (22.8625, -19.6822) -> (22.8603, 19.6878) centre (1.379, 0.0016) ccw
  line L17 (50.7998, 28.5794) -> (22.8598, 28.5778)
  circle A4 centre (26.67, 24.768) radius 1.4
  circle A5 centre (26.6728, -24.762) radius 1.4
  line L18 (22.8626, -20.9522) -> (24.1326, -20.9521)
  line L19 (22.8625, -19.6822) -> (22.8626, -20.9522)
  line L20 (24.1326, -20.9521) -> (24.1327, -23.4921)
  line L21 (24.1327, -23.4921) -> (22.8627, -23.4922)
  line L22 (22.8627, -23.4922) -> (22.863, -28.5722)
  line L23 (22.863, -28.5722) -> (50.803, -28.5706)
  line L24 (50.803, -28.5706) -> (50.7998, 28.5794)
  line L25 (-50.797, -28.5764) -> (-50.8002, 28.5736)
  point P0 (0, 0)
  constraints: 52 end point, 6 centre point, 4 point on circle, 66 other
extrude "Extrusion55" cut sketch "Sketch58" along normal blind 1.1 contours L0 L1 L2 L3 L4 L5 A1 L6 L7 L8 L9 L10 L11 L25 | A0 | A2 | L13 L14 L17 L24 L23 L22 L21 L20 L18 L19 A3 L16 L15 L12 | A4 | A5
sketch "Sketch59" plane through (-30.17, -28.575, -22) normal (0, 1, 0) x (1, 0, 0)
  line L0 (60.34, -22) -> (60.34, 0) projected
  line L1 (0, 0) -> (60.34, 0)
  line L2 (60.34, 0) -> (60.34, -4)
  line L3 (60.34, -4) -> (0, -4)
  line L4 (0, -4) -> (0, 0)
  line L5 (0, -22) -> (0, 0) projected
  line L6 (0, -5) -> (60.34, -5)
  line L7 (60.34, -5) -> (60.34, -15)
  line L8 (60.34, -15) -> (0, -15)
  line L9 (0, -15) -> (0, -5)
  line L10 (0, -16) -> (60.34, -16)
  line L11 (60.34, -16) -> (60.34, -17)
  line L12 (60.34, -17) -> (0, -17)
  line L13 (0, -17) -> (0, -16)
  line L14 (7.8, -17) -> (52.54, -17)
  line L15 (52.54, -17) -> (52.54, -18)
  line L16 (52.54, -18) -> (7.8, -18)
  line L17 (7.8, -18) -> (7.8, -17)
  line L18 (7.8, -22) -> (7.8, -23) projected
  line L19 (52.54, -22) -> (52.54, -23) projected
  point P0 (30.17, -22)
  dimension "d424" = 4
  dimension "d429" = 1
  dimension "d430" = 10
  dimension "d433" = 1
  dimension "d434" = 1
  dimension "d435" = 1
  constraints: 32 end point, 8 parallel, 6 point on line, 4 horizontal, 4 perpendicular, 2 collinear
  measures "d424" distance between parallel lines of L1 L3
  measures "d429" distance between parallel lines of L3 L6
  measures "d430" distance between parallel lines of L6 L8
  measures "d433" distance between parallel lines of L8 L10
  measures "d434" distance between parallel lines of L10 L12
  measures "d435" distance between parallel lines of L16 L14
extrude "Extrusion56" add sketch "Sketch59" along normal blind 1 contours L12 L5 L10 L0 | L15 L16 L17 L12 | L8 L5 L6 L0 | L3 L4 L1 L0
sketch "Sketch60" plane through (-30.17, -28.575, -22) normal (0, -1, 0) x (1, 0, 0)
  arc A0 (32.1272, 16) -> (33.3054, 18) centre (30.17, 18.5) ccw projected
  circle A1 centre (30.17, 18.5) radius 3.175
  arc A2 (32.9683, 5) -> (27.3717, 5) centre (30.17, 6.5) ccw projected
  line L0 (32.9683, 5) -> (27.3717, 5) projected
  circle A3 centre (30.17, 6.5) radius 3.175
  point P0 (30.17, 22)
  constraints: 2 centre point, 2 coincident, 2 concentric
extrude "Extrusion57" add sketch "Sketch60" along normal blind 1
sketch "Sketch61" plane through (-30.17, 31.575, 9) normal (0, 1, 0) x (1, 0, 0)
  line L0 (60.34, 9) -> (0, 9) projected
  line L1 (0, 9) -> (0, 0) projected
  circle A0 centre (4, 5) radius 1.4
  line L2 (60.34, 0) -> (0, 0) projected
  line L3 (50.17, 6) -> (10.17, 6) projected
  line L4 (30.17, 0) -> (30.17, 3.6) construction
  circle A1 centre (56.34, 5) radius 1.4
  point P0 (10.17, 9)
  point P1 (30.17, 9)
  dimension "d438" = 2.8
  dimension "d439" = 4
  dimension "d440" = 4
  constraints: 2 centre point, 2 end point, 1 midpoint, 1 perpendicular, 1 symmetric about line, 1 other
  measures "d438" diameter of A0
  measures "d439" distance from line of L1 A0.centre
  measures "d440" distance from line of L0 A0.centre
extrude "Extrusion58" cut sketch "Sketch61" against normal blind 5
thread "Thread1" size "M3x0.5" class "6H" standard "ANSI Metric M Profile" full length
thread "Thread2" size "M3x0.5" class "6H" standard "ANSI Metric M Profile" full length
body "Solid1"
